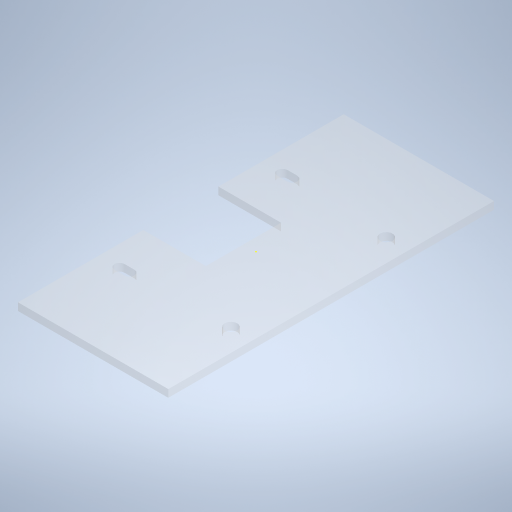
# Autodesk Inventor part: 발받침대받침옆판
Saved by Autodesk Inventor 2024 (Build 280153000, 153)
## iProperties
Created: 2024-04-10
Part Number: 발받침대받침옆판
Material: PMMA 플라스틱
Document SubType Name: Modeling
Designer: kkamin5
Mass: 39.204 g
Surface Area: 149 cm^2
Volume: 33 cm^3
Density: 1.188 g/cm^3
Appearance: 폴리카보네이트 - 선명
Author: kkamin5
Autodesk Inventor part; units mm, degrees
ref_plane "YZ Plane" through (0, 0, 0) normal (1, 0, 0) x (0, 1, 0)
ref_plane "XZ Plane" through (0, 0, 0) normal (0, 1, 0) x (-1, 0, 0)
ref_plane "XY Plane" through (0, 0, 0) normal (0, 0, 1) x (1, 0, 0)
sketch "스케치1" plane through (0, 0, 0) normal (0, 1, 0) x (-1, 0, 0)
  line L0 (30, 65) -> (-30, 65)
  line L1 (-30, 65) -> (-30, -65)
  line L2 (-30, -65) -> (30, -65)
  line L3 (30, -65) -> (30, 65)
  point P0 (0, 0)
  dimension "d0" = 130
  dimension "d1" = 60
  dimension "d2" = 30
  dimension "d3" = 65
  constraints: 8 end point, 2 parallel, 1 horizontal, 1 perpendicular
  measures "d0" distance of L0.end L1.end
  measures "d1" distance of L1.end L2.end
  measures "d2" distance from line of point (0, 0) L3
  measures "d3" distance from line of point (0, 0) L0
extrude "돌출1" add sketch "스케치1" along normal blind 3
sketch "스케치2" plane through (0, 3, 0) normal (0, 1, 0) x (1, 0, 0)
  point P0 (0, 0)
sketch "스케치3" plane through (0, 3, 0) normal (0, 1, 0) x (1, 0, 0)
  line L0 (66.1835, 32.5) -> (-80.6968, 32.5)
  line L1 (66.1835, -32.5) -> (-80.6968, -32.5)
  line L2 (-30, -65) -> (30, -65) projected
  line L3 (30, 65) -> (-30, 65) projected
  line L4 (-22, 32.5) -> (-18, 32.5) construction
  line L5 (-22, 30.5) -> (-18, 30.5)
  line L6 (-18, 34.5) -> (-22, 34.5)
  arc A0 (-22, 34.5) -> (-22, 30.5) centre (-22, 32.5) ccw
  arc A1 (-18, 30.5) -> (-18, 34.5) centre (-18, 32.5) ccw
  line L7 (-30, 65) -> (-30, -65) projected
  line L8 (-22, -32.5) -> (-18, -32.5) construction
  line L9 (-22, -34.5) -> (-18, -34.5)
  line L10 (-18, -30.5) -> (-22, -30.5)
  arc A2 (-22, -30.5) -> (-22, -34.5) centre (-22, -32.5) ccw
  arc A3 (-18, -34.5) -> (-18, -30.5) centre (-18, -32.5) ccw
  line L11 (30, -65) -> (30, 65) projected
  circle A4 centre (21, 31) radius 2.5
  circle A5 centre (21, -31) radius 2.5
  line L12 (-30, -15) -> (-5, -15)
  line L13 (-5, -15) -> (-5, 15)
  line L14 (-5, 15) -> (-30, 15)
  line L15 (-30, 15) -> (-30, -15)
  line L16 (-30, -15) -> (-5, 15) construction
  line L17 (-5, -15) -> (-30, 15) construction
  point P0 (0, 0)
  point P1 (-20, 32.5)
  point P2 (-20, -32.5)
  point P3 (-17.5, 0)
  point P4 (-30, 15)
  dimension "d6" = 32.5
  dimension "d7" = 32.5
  dimension "d8" = 4
  dimension "d9" = 4
  dimension "d11" = 4
  dimension "d17" = 10
  dimension "d18" = 10
  dimension "d33" = 5
  dimension "d34" = 5
  dimension "d35" = 62
  dimension "d36" = 31
  dimension "d37" = 9
  dimension "d38" = 0
  dimension "d39" = 25
  dimension "d40" = 30
  dimension "d41" = 0
  dimension "d42" = 12.5
  dimension "d43" = 4
  constraints: 32 end point, 8 point on circle, 8 tangent, 6 centre point, 4 midpoint, 4 parallel, 4 point on line, 3 horizontal, 1 perpendicular
  measures "d6" distance between parallel lines of L2 L1
  measures "d7" distance between parallel lines of L3 L0
  measures "d8" distance of L4.start L4.end
  measures "d9" diameter of A1
  measures "d11" diameter of A3
  measures "d17" distance from line of L7 point (-20, -32.5)
  measures "d18" distance from line of L7 point (-20, 32.5)
  measures "d33" diameter of A4
  measures "d34" diameter of A5
  measures "d35" distance of A4.centre A5.centre
  measures "d36" vertical distance of point (0, 0) A5.centre
  measures "d37" distance from line of L11 A5.centre
  measures "d38" horizontal distance of A5.centre A4.centre
  measures "d39" distance of L14.end L13.end
  measures "d40" distance of L13.end L12.end
  measures "d41" vertical distance of point (0, 0) point (-17.5, 0)
  measures "d42" distance from line of L7 point (-17.5, 0)
  measures "d43" distance of L10.start L10.end
extrude "돌출2" cut sketch "스케치3" against normal blind 10 contours A4 L0 | L0 A4 | A5 L1 | L1 A5 | A1 L5 A0 L0 | L0 A0 L6 A1 | A3 L9 A2 L1 | L1 A2 L10 A3 | L14 L13 L12 L7
equation "\"d3\" = 0.5 * d0"
equation "\"d36\" = 0.5 * d35"
equation "\"d42\" = 0.5 * d39"
